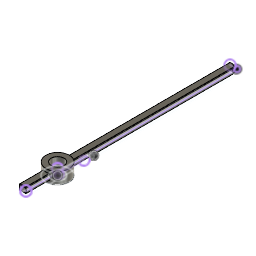
Naciskacz_colletive (Autodesk Fusion 360 design; units mm, degrees)
part number: 2026-02-12-15-13-30-636
Autodesk Fusion 360 part; units mm, degrees
note: some values were not read from the file. Set by a fixed rule: which sketch regions a step uses.
sketch "Szkic1" plane through (0, 0, 0) normal (0, 0, 1) x (1, 0, 0)
  circle A0 centre (0, 0) radius 5.5
  line L0 (-3, 150) -> (3, 150)
  line L1 (3, 150) -> (3, -30)
  line L2 (3, -30) -> (-3, -30)
  line L3 (-3, -30) -> (-3, 150)
  line L4 (0, 1.75) -> (0, 22.5)
  circle A1 centre (0, 0) radius 10
  dimension "d7" = 11
  dimension "d8" = 30
  dimension "d10" = 6
  dimension "d11" = 180
  dimension "d12" = 20
  constraint coincident A0.centre A1.centre
  constraint horizontal L0
  constraint vertical L1
  constraint horizontal L2
  constraint vertical L3
  constraint symmetric L1.end L2.end L4
  measures "d7" diameter of A0
  measures "d8" distance of A0.centre L2
  measures "d10" distance of L1 L3
  measures "d11" distance of L0.end L1.end
  measures "d12" diameter of A1
extrude "Wyciągnięcie proste1" add sketch "Szkic1" along normal blind 10 contours A0 L1 A1 | A0 L1 L4 A1 | A0 L1 L3 A1 | A0 L3 L4 A1 | A0 L3 A1
extrude "Wyciągnięcie proste2" add sketch "Szkic1" along normal blind 5 from surface at 2.5 contours L0 L1 L3 A1 | L1 L2 L3 A1
ref_plane "Płaszczyzna konstrukcyjna1" through (0, -19.7697, 5) normal (0, 0, 1) x (1, 0, 0)
sketch "Szkic2" plane through (0, 0, 5) normal (0, 0, 1) x (1, 0, 0)
  circle A0 centre (6, 25) radius 2.5
  line L0 (4.9, 22.755) -> (3, 22.755)
  line L1 (3, 22.755) -> (3, 27.245)
  line L2 (3, 27.245) -> (4.9, 27.245)
  line L3 (4.9, 27.245) -> (4.9, 22.755)
  line L4 (3, 150) -> (3, -30)
  line L5 (6, 25) -> (3, 25)
  line L6 (7.25, 22.8349) -> (7.25, 27.1651)
  circle A1 centre (6, 25) radius 1.75
  line L7 (7.7321, 24.75) -> (6, 24.75)
  line L8 (6, 24.75) -> (6, 25.25)
  line L9 (6, 25.25) -> (7.7321, 25.25)
  line L10 (7.7321, 25.25) -> (7.7321, 24.75)
  line L11 (-3, 150) -> (3, 150)
  dimension "d18" = 5
  dimension "d19" = 1.25
  dimension "d20" = 3.5
  dimension "d21" = 0.5
  dimension "d22" = 25
  dimension "d23" = 125
  dimension "d24" = 1.1
  dimension "d25" = 3
  constraint horizontal L0
  constraint vertical L1
  constraint horizontal L2
  constraint vertical L3
  constraint coincident A0 L0.start
  constraint collinear L1 L4
  constraint coincident A0.centre L5.start
  constraint coincident L1 L5.end
  constraint perpendicular L1 L5
  constraint symmetric L0 L2 L5
  constraint coincident A0 L6.start
  constraint coincident A0 L6.end
  constraint vertical L6
  constraint concentric A0 A1
  constraint horizontal L7
  constraint vertical L8
  constraint horizontal L9
  constraint vertical L10
  constraint coincident A1 L7.start
  constraint symmetric L5 L7 L9
  constraint coincident A0.centre L8
  measures "d18" diameter of A0
  measures "d19" distance of A0.centre L6
  measures "d20" diameter of A1
  measures "d21" distance of L7 L9
  measures "d22" vertical distance of L5.end origin
  measures "d23" distance of L5 L11
  measures "d24" distance of L3 A0.centre
  measures "d25" distance of A0.centre L1
revolve "Obrót1" add sketch "Szkic2" angle 360 about axis through (6, 25, 5) along (-1, 0, 0) contours A0 L3 L6 A1 | A0 L0 L1 L4 L5 | A0 L3 L5 A1 picked at (5.1557, 22.9188) picked at (4.6078, 23.2377)
extrude "Wyciągnięcie proste3" cut sketch "Szkic2" along normal through all and the other way through all contours L6 L7 L8 L9
pattern_circular "Szyk kołowy1" count 2 over 90 about axis through (6, 25, 5) along (-1, 0, 0) of "Wyciągnięcie proste3"
fillet "Zaokrąglenie1" radius 0.5 15 edges at (3, 79.7697, 7.5) (-3, 79.7697, 7.5) (3, 79.7697, 2.5) (-3, 79.7697, 2.5) (3, -19.7697, 7.5) (-3, -19.7697, 7.5) (3, -19.7697, 2.5) (-3, -19.7697, 2.5) (-3, -30, 5) (0, -30, 7.5) (3, -30, 5) (0, -30, 2.5) (0, 150, 7.5) (-3, 150, 5) (0, 150, 2.5)
fillet "Zaokrąglenie1" radius 4 1 edges at (3, 150, 5)
